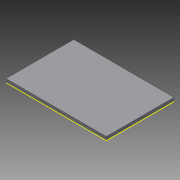
# Autodesk Inventor part: Deckel
Saved by Autodesk Inventor 2014 (Build 180170000, 170)
## iProperties
Created: 2016-07-27
Part Number: Deckel
Material: Generisch
Document SubType Name: Modeling
Designer: cem
Density: 1 g/cm^3
Appearance: Beige
Author: cem
Autodesk Inventor part; units mm, degrees
ref_plane "YZ Plane" through (0, 0, 0) normal (1, 0, 0) x (0, 1, 0)
ref_plane "XZ Plane" through (0, 0, 0) normal (0, 1, 0) x (-1, 0, 0)
ref_plane "XY Plane" through (0, 0, 0) normal (0, 0, 1) x (1, 0, 0)
sketch "SkizzeDeckel" plane through (0, 0, 0) normal (0, 0, 1) x (1, 0, 0)
  line L0 (-30.17, 0) -> (30.17, 0) projected
  line L1 (0, -20.37) -> (0, 20.37) projected
  line L2 (21.55, -14.55) -> (-21.55, -14.55) projected
  line L3 (-21.55, 14.55) -> (21.55, 14.55)
  line L4 (21.55, 14.55) -> (21.55, -14.55)
  line L5 (21.55, -14.55) -> (-21.55, -14.55)
  line L6 (-21.55, -14.55) -> (-21.55, 14.55)
  line L7 (-21.55, -14.55) -> (-21.55, -9.7) projected
  point P0 (0, 0)
  constraints: 8 end point, 2 collinear, 2 parallel, 1 horizontal, 1 perpendicular, 2 other
extrude "Deckel" add sketch "SkizzeDeckel" along normal blind 1.5
sketch "SkizzeStecker" plane through (0, 0, 0) normal (0, 0, -1) x (-1, 0, 0)
  line L0 (-21.55, 14.55) -> (-21.55, -14.55) projected
  line L1 (21.55, -14.55) -> (21.55, 14.55) projected
  line L2 (-20.05, -12.7) -> (-20.05, 12.7) projected
  line L3 (-21.55, -12.7) -> (-20.05, -12.7) projected
  line L4 (-21.55, 12.7) -> (-21.55, -12.7) projected
  line L5 (-21.55, 12.7) -> (-20.05, 12.7) projected
  line L6 (20.05, 9.7) -> (20.05, -9.7) projected
  line L7 (21.55, 9.7) -> (20.05, 9.7) projected
  line L8 (21.55, -9.7) -> (21.55, 9.7) projected
  line L9 (21.55, -9.7) -> (20.05, -9.7) projected
  line L10 (-21.55, -12.65) -> (-18.05, -12.65)
  line L11 (-18.05, -12.65) -> (-18.05, 12.65)
  line L12 (-18.05, 12.65) -> (-21.55, 12.65)
  line L13 (-21.55, 12.65) -> (-21.55, -12.65)
  line L14 (30.17, 0) -> (-30.17, 0) projected
  line L15 (21.55, 9.65) -> (18.05, 9.65)
  line L16 (18.05, 9.65) -> (18.05, -9.65)
  line L17 (18.05, -9.65) -> (21.55, -9.65)
  line L18 (21.55, -9.65) -> (21.55, 9.65)
  point P0 (0, 0)
  dimension "d2" = 0.05
  dimension "d3" = 3.5
  dimension "d4" = 0.05
  constraints: 16 end point, 5 parallel, 2 collinear, 2 horizontal, 2 perpendicular, 2 other
  measures "d2" distance between parallel lines of L5 L12
  measures "d3" distance between parallel lines of L11 L4
  measures "d4" distance between parallel lines of L15 L7
ref_plane "Arbeitsebene1" through (14.6, -2.6, -1.5) normal (0, 0, 1) x (1, 0, 0)
extrude "Stecker" add sketch "SkizzeStecker" along normal up to surface (1.5 mm away) contours L12 L2 L14 L0 | L14 L2 L10 L0 | L12 L11 L14 L2 | L14 L11 L10 L2 | L17 L6 L14 L1 | L14 L6 L15 L1 | L17 L16 L14 L6 | L14 L16 L15 L6
sketch "SkizzeLippe" plane through (0, 0, 0) normal (0, 0, -1) x (-1, 0, 0)
  line L0 (30.17, 0) -> (-30.17, 0) projected
  line L1 (0, -20.37) -> (0, 20.37) projected
  line L2 (-20.7, 13.7) -> (20.7, 13.7)
  line L3 (20.7, 13.7) -> (20.7, -13.7)
  line L4 (20.7, -13.7) -> (-20.7, -13.7)
  line L5 (-20.7, -13.7) -> (-20.7, 13.7)
  line L6 (-20.75, -12.7) -> (-20.75, -13.75) projected
  line L7 (-20.75, -13.75) -> (20.75, -13.75) projected
  line L8 (20.75, 9.7) -> (20.75, 13.75) projected
  line L9 (20.75, 13.75) -> (7.5, 13.75) projected
  point P0 (0, 0)
  dimension "d7" = 0.05
  dimension "d8" = 0.05
  constraints: 8 end point, 2 parallel, 1 horizontal, 1 perpendicular, 2 other
  measures "d7" distance between parallel lines of L8 L3
  measures "d8" distance between parallel lines of L9 L2
ref_plane "LippeEbene" through (0, 0, -0.55) normal (0, 0, 1) x (1, 0, 0)
extrude "Lippe" add sketch "SkizzeLippe" along normal up to surface (0.55 mm away)
sketch "SkizzeSchnapperarm" plane through (20.7, -13.7, -0.55) normal (0, 0, -1) x (-1, 0, 0)
  line L0 (34.1, 0.65) -> (29.6, 0.65) projected
  line L1 (29.65, 0.7) -> (34.05, 0.7)
  line L2 (34.05, 0.7) -> (34.05, 2.2)
  line L3 (34.05, 2.2) -> (29.65, 2.2)
  line L4 (29.65, 2.2) -> (29.65, 0.7)
  line L5 (29.6, -0.85) -> (29.6, 0.65) projected
  line L6 (34.1, -0.85) -> (34.1, 0.65) projected
  line L7 (31.85, -1.277) -> (31.85, 1.312) construction
  point P0 (20.7, 13.7)
  point P1 (31.85, 0.65)
  dimension "d11" = 0.05
  dimension "d12" = 1.5
  dimension "d13" = 0.05
  constraints: 10 end point, 3 parallel, 1 horizontal, 1 midpoint, 1 perpendicular, 1 point on line, 1 other
  measures "d11" distance between parallel lines of L0 L1
  measures "d12" distance between parallel lines of L1 L3
  measures "d13" distance between parallel lines of L4 L5
ref_plane "EbeneSchnapper" through (-8.9, -14.55, -3.85) normal (0, 0, 1) x (1, 0, 0)
extrude "Schnapperarm" add sketch "SkizzeSchnapperarm" along normal up to surface (3.3 mm away)
sketch "SkizzeSchnapper" plane through (-13.35, -13, -0.55) normal (0, -1, 0) x (1, 0, 0)
  line L0 (4.4, -3.3) -> (0, -3.3) projected
  line L1 (4.4, 0) -> (4.4, -3.3) projected
  line L2 (-0.05, -1.85) -> (4.45, -1.85) projected
  line L3 (-0.05, -3.45) -> (-0.05, -1.85) projected
  line L4 (4.45, -3.45) -> (-0.05, -3.45) projected
  line L5 (4.45, -1.85) -> (4.45, -3.45) projected
  line L6 (0, -3.3) -> (4.4, -3.3)
  line L7 (4.4, -3.3) -> (4.4, -1.9)
  line L8 (4.4, -1.9) -> (0, -1.9)
  line L9 (0, -1.9) -> (0, -3.3)
  point P0 (13.35, 0.55)
  dimension "d16" = 0.05
  constraints: 8 end point, 2 parallel, 1 horizontal, 1 perpendicular, 1 point on line
  measures "d16" distance between parallel lines of L2 L8
ref_plane "EbeneSchnapperTiefe" through (21.55, -13.8, -8.8) normal (0, -1, 0) x (-1, 0, 0)
extrude "Schnapper" add sketch "SkizzeSchnapper" along normal up to surface (0.8 mm away) contours L0 L9 L8 L1
chamfer "FaseSchnapper" distance 1 distance2 1.25 1 edges at (-11.15, -13.8, -3.85) measured on face at (-11.15, -13.3, -3.85)
draft "FlächenverjüngungSchnapper" angle 12 pull direction (0, 0, -1) fixed plane through (-2.9833, 3.6, -0.55) normal (0, 0, -1) faces at (-11.8833, -11.5, -1.65)
mirror "SpiegelnSchnapper1" about plane through (0, 0, 0) normal (0, 1, 0) of "Schnapperarm", "Schnapper", "FaseSchnapper", "FlächenverjüngungSchnapper"
mirror "SpiegelnSchnapper2" about plane through (0, 0, 0) normal (1, 0, 0) of "Schnapperarm", "Schnapper", "FaseSchnapper", "FlächenverjüngungSchnapper", "SpiegelnSchnapper1"
sketch "Skizze6" plane through (0, 0, 0) normal (0, 0, -1) x (-1, 0, 0)
  line L0 (21.55, 14.55) -> (-21.55, 14.55)
  line L1 (7.5, 13.75) -> (7.5, 14.55)
  line L2 (-1, 14.55) -> (-1, 13.75)
  line L3 (-1, 13.05) -> (-1, 13.75)
  line L4 (7.5, 13.75) -> (7.5, 13.05)
  line L5 (0, 13.05) -> (-1, 13.05)
  line L6 (0, 13.05) -> (6.5, 13.05)
  line L7 (7.5, 13.05) -> (6.5, 13.05)
  line L8 (-0.95, 13.05) -> (7.45, 13.05)
  line L9 (7.45, 13.05) -> (7.45, 14.55)
  line L10 (7.45, 14.55) -> (-0.95, 14.55)
  line L11 (-0.95, 14.55) -> (-0.95, 13.05)
  line L12 (3.25, 12.1908) -> (3.25, 15.4162) construction
  point P0 (0, 0)
  point P1 (3.25, 13.05)
extrude "USB" add sketch "Skizze6" along normal blind 1.9 contours L9 L7 L6 L5 L11 L0
sketch "Skizze8" plane through (0, 0, 1.5) normal (0, 0, 1) x (1, 0, 0)
  line L0 (-21.55, 14.55) -> (-21.55, -14.55) projected
  line L1 (-8.9054, 0.1316) -> (-2.5661, -13.4631)
  line L2 (-8.9054, 0.1316) -> (6.0946, 0.1316) construction
  line L3 (-15.55, 2.55) -> (-9.2107, -11.0446)
  line L4 (-9.2107, -11.0446) -> (-20.0864, -16.116)
  line L5 (-15.55, 2.55) -> (-0.55, 2.55) construction
  line L6 (-15.55, 2.55) -> (-8.9054, 0.1316)
  line L7 (-21.55, -14.55) -> (21.55, -14.55) projected
  line L8 (21.55, 14.55) -> (-21.55, 14.55) projected
  line L9 (-20.0864, -16.116) -> (-17.9733, -20.6476)
  line L10 (-2.5661, -13.4631) -> (-17.9733, -20.6476)
  line L11 (-19.5368, 4.0011) -> (-13.1975, -9.5935)
  line L12 (-26.1814, 6.4195) -> (-19.8421, -7.1751)
  line L13 (-19.8421, -7.1751) -> (-30.7178, -12.2465)
  line L14 (-26.1814, 6.4195) -> (-19.5368, 4.0011)
  line L15 (-30.7178, -12.2465) -> (-28.6047, -16.7781)
  line L16 (-13.1975, -9.5935) -> (-28.6047, -16.7781)
  line L17 (-4.897, -14.55) -> (-16.728, -14.55)
  line L18 (-21.55, 4.7338) -> (-21.55, -3.5126)
  line L19 (-21.55, -7.9715) -> (-21.55, -13.4884)
  point P0 (0, 0)
  dimension "d28" = 65
  dimension "d32" = 65
  dimension "d37" = 5
  dimension "d38" = 15
  dimension "d39" = 12
  dimension "d40" = 5
  dimension "d41" = 6
  dimension "d42" = 12
  dimension "d43" = 5
  dimension "d44" = 15
  dimension "d45" = 5
  dimension "d46" = 12
  dimension "d48" = 3
  dimension "d49" = 3
  constraints: 34 end point, 12 point on line, 6 perpendicular, 4 equal length, 2 horizontal, 1 parallel
  measures "d28" angle of L1 L2
  measures "d32" angle of L3 L5
  measures "d37" distance between parallel lines of L3 L1
  measures "d38" distance from line of L4 L3.start
  measures "d39" distance between parallel lines of L5 L8
  measures "d40" distance between parallel lines of L10 L4
  measures "d41" distance from line of L3.start L0
  measures "d42" distance between parallel lines of L9 L3
  measures "d43" distance between parallel lines of L12 L11
  measures "d44" distance from line of L13 L14.start
  measures "d45" distance between parallel lines of L16 L13
  measures "d46" distance between parallel lines of L15 L12
  measures "d48" distance between parallel lines of L3 L11
  measures "d49" distance between parallel lines of L4 L16
extrude "Extrusion8" add sketch "Skizze8" along normal blind 0.5 contours L14 L11 L16 L0 L13 L12 | L1 L10 L7 L4 L3 L6
fillet "Rundung1" radius 1 10 edges at (-12.2277, 1.3408, 2) (-12.3804, -4.2473, 2) (-5.7357, -6.6658, 2) (-12.9694, -12.7973, 2) (-3.7316, -14.0065, 2) (-17.3738, -11.541, 2) (-20.6961, -5.3438, 2) (-20.6961, -7.5733, 2) (-16.3671, -2.7962, 2) (-20.5434, 4.3674, 2)
